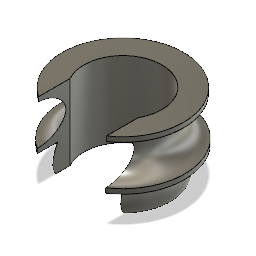
PCBmillFoot v2 (Autodesk Fusion 360 design; units mm, degrees)
Autodesk Fusion 360 part; units mm, degrees
sketch "Sketch1" plane through (0, 0, 0) normal (1, 0, 0) x (0, 0, -1)
  line L0 (12.7405, 0.5) -> (-12.7405, 0.5)
  line L1 (-12.7405, 0.5) -> (-12.7405, -0.5)
  line L2 (-12.7405, -0.5) -> (12.7405, -0.5)
  line L3 (12.7405, -0.5) -> (12.7405, 0.5)
  line L4 (12.7405, 0.5) -> (-12.7405, -0.5) construction
  line L5 (-12.7405, 0.5) -> (12.7405, -0.5) construction
  line L6 (12.5, 9.58) -> (-12.5, 9.58)
  line L7 (12.5, 8.58) -> (12.5, 9.58)
  line L8 (12.5, 9.58) -> (-12.5, 8.58) construction
  line L9 (-12.5, 9.58) -> (12.5, 8.58) construction
  line L10 (-12.5, 8.58) -> (12.5, 8.58)
  line L11 (-12.5, 9.58) -> (-12.5, 8.58)
  arc A0 (-12.7405, 0.5) -> (-12.5, 8.58) centre (-12.5, 4.5364) ccw
  arc A1 (12.5, 8.58) -> (12.7405, 0.5) centre (12.582, 4.5389) ccw
  line L12 (-8.4582, 4.4161) -> (8.5418, 4.4186) construction
  line L13 (0, 9.08) -> (0, 0) construction
  line L14 (-9.5, -0.5) -> (-10.8653, -4.25)
  line L15 (-10.8653, -4.25) -> (-9.75, -6)
  spline S0 degree 2 poles (-9.5, -0.5) (-10.8653, -4.25) (-9.75, -6) knots 0 0 0 1 1 1
  line L16 (9.5, -0.5) -> (10.8653, -4.25)
  line L17 (10.8653, -4.25) -> (9.75, -6)
  spline S1 degree 2 poles (9.5, -0.5) (10.8653, -4.25) (9.75, -6) knots 0 0 0 1 1 1
  line L18 (-9.75, -6) -> (9.75, -6)
  line L19 (0, -6) -> (0, 0) construction
  line L20 (-10.8653, -4.25) -> (10.8653, -4.25) construction
  line L21 (0, 9.58) -> (0, -6)
  dimension "d2" = 1
  dimension "d3" = 25
  dimension "d4" = 1
  dimension "d5" = 10.08
  dimension "d6" = 17
  dimension "d7" = 19
  dimension "d8" = 19.5
  dimension "d10" = 5.5
  dimension "d11" = 20.5
  dimension "d12" = 1.75
  measures "d5" distance of L2 L6
  measures "d12" distance of L18 L20
revolve "Revolve1" add sketch "Sketch1" angle 360 about axis through (0, 9.58, 0) along (0, -1, 0) contours L0 L1 L2 A0 L21 | L0 L10 A0 L21 | L6 L10 L11 L21 | L2 S0 L18 L21
sketch "Sketch2" plane through (0, -6, 0) normal (0, -1, 0) x (1, 0, 0)
  circle A0 centre (0, 0) radius 9.75
  circle A1 centre (0, 0) radius 8
  circle A2 centre (0, 0) radius 12.5
  line L0 (-7, 3.873) -> (-7, 10.6452)
  line L1 (7, 3.873) -> (7, 10.6452)
  circle A3 centre (0, 0) radius 12.7405
  dimension "d14" = 16
  dimension "d15" = 14
  measures "d14" diameter of A1
  measures "d15" distance of L0 L1
extrude "Extrude1" cut sketch "Sketch2" against normal up to surface (15.58 mm away) contours A0 A1 L0 L1 | A0 A2 L0 L1 | A1 | A2 L0 L1 A3 picked at (6.1916, 6.7325) picked at (0.8533, 11.5288) picked at (-6.4632, 10.7599)
